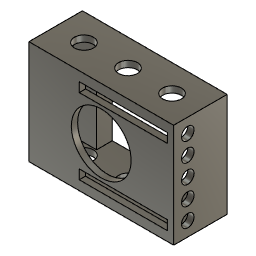
esp32 Box (Autodesk Fusion 360 design; units mm, degrees)
Autodesk Fusion 360 part; units mm, degrees
note: some values were not read from the file. Set by a fixed rule: which sketch regions a step uses.
sketch "Skizze1" plane through (0, 0, 0) normal (0, 1, 0) x (1, 0, 0)
  line L0 (0, 0) -> (46, 0)
  line L1 (46, 0) -> (46, -33)
  line L2 (46, -33) -> (0, -33)
  line L3 (0, -33) -> (0, 0)
  line L4 (2, -2) -> (44, -2)
  line L5 (44, -2) -> (44, -31)
  line L6 (44, -31) -> (2, -31)
  line L7 (2, -31) -> (2, -2)
  dimension "d1" = 46
  dimension "d2" = 33
  dimension "d3" = 2
  constraint horizontal L0
  constraint vertical L1
  constraint horizontal L2
  constraint vertical L3
  constraint coincident L0.start L3.end
  measures "d1" distance of L0.start L0.end
  measures "d2" distance of L0.start L2.end
extrude "Extrusion1" add sketch "Skizze1" against normal blind 2 contours L0 L1 L2 L3 | L4 L5 L6 L7
extrude "Extrusion2" add sketch "Skizze1" along normal blind 15
sketch "Skizze2" plane through (0, 0, 0) normal (0, 1, 0) x (1, 0, 0)
sketch "Skizze3" plane through (0, 15, 0) normal (0, 1, 0) x (-1, 0, 0)
  line L0 (-44, 31) -> (-2, 31)
  line L1 (-2, 31) -> (-2, 2)
  line L2 (-2, 2) -> (-44, 2)
  line L3 (-44, 2) -> (-44, 31)
  line L4 (0, 33) -> (-46, 33)
  line L5 (-46, 33) -> (-46, 0)
  line L6 (-46, 0) -> (0, 0)
  line L7 (0, 0) -> (0, 33)
  line L8 (-2, 31) -> (-9.5, 31)
  line L9 (-9.5, 31) -> (-9.5, 2)
  line L10 (-9.5, 2) -> (-2, 2)
  line L11 (-2, 2) -> (-2, 31)
  dimension "d8" = 7.5
  constraint horizontal L8
  constraint vertical L9
  constraint horizontal L10
  constraint vertical L11
  constraint coincident L0.end L1.start
  measures "d8" distance of L0.end L8.end
extrude "Extrusion3" add sketch "Skizze3" against normal blind 5 contours L0 L1 L2 L8 L9 L10 L11
sketch "Skizze4" plane through (0, -2, 0) normal (0, -1, 0) x (1, 0, 0)
  line L0 (46, 33) -> (0, 33)
  line L1 (0, 33) -> (0, 0)
  line L2 (0, 0) -> (46, 0)
  line L3 (46, 0) -> (46, 33)
  line L4 (46, 33) -> (16, 33)
  line L5 (16, 33) -> (16, 0)
  line L6 (16, 0) -> (46, 0)
  line L7 (46, 0) -> (46, 33)
  line L8 (16, 33) -> (46, 33)
  line L9 (16, 30) -> (16, 33)
  line L10 (16, 0) -> (46, 0)
  line L11 (46, 0) -> (46, 3)
  line L12 (46, 3) -> (16, 3)
  line L13 (16, 3) -> (16, 0)
  line L14 (16, 3) -> (46, 3)
  line L15 (46, 3) -> (46, 6)
  line L16 (46, 6) -> (16, 6)
  line L17 (16, 6) -> (16, 3)
  line L18 (0, 33) -> (46, 0)
  line L19 (46, 33) -> (0, 0)
  circle A0 centre (23, 16.5) radius 9.5
  line L20 (44, 35) -> (44, -3)
  line L21 (16, 30) -> (44, 30)
  line L22 (44, 30) -> (44, 27)
  line L23 (44, 27) -> (16, 27)
  line L24 (16, 27) -> (16, 30)
  dimension "d12" = 3
  constraint horizontal L4
  constraint vertical L5
  constraint horizontal L6
  constraint vertical L7
  constraint coincident L2 L5.end
  constraint coincident L0.start L3.end
  constraint horizontal L8
  constraint vertical L9
  constraint horizontal L10
  constraint vertical L11
  constraint horizontal L12
  constraint vertical L13
  constraint coincident L3 L11.end
  constraint horizontal L14
  constraint vertical L15
  constraint horizontal L16
  constraint vertical L17
  constraint coincident L0.end L1.start
  constraint coincident L1.end L2.start
  constraint midpoint L18 A0.centre
  constraint perpendicular L10 L20
  constraint horizontal L21
  constraint vertical L22
  constraint horizontal L23
  constraint vertical L24
  constraint coincident L20 L22.end
  measures "d12" distance of L12.end L16.end
extrude "Extrusion4" cut sketch "Skizze4" against normal blind 6 contours L5 L19 L21 L23 L24 | L5 L18 A0 | L5 L18 L19 A0 | L19 L20 L21 L22 L23 | L5 L19 A0 | L5 L18 L19 | L5 L18 L19 A0 | L5 L12 L14 L16 L17 L18 | L5 L18 L19 A0 | L18 L19 A0 | L12 L14 L16 L18 L20
sketch "Skizze5" plane through (0, 0, 0) normal (0, 0, -1) x (1, 0, 0)
  line L0 (46, -15) -> (46, 2)
  line L1 (46, 2) -> (0, 2)
  line L2 (0, 2) -> (0, -15)
  line L3 (0, -15) -> (46, -15)
  line L4 (46, -15) -> (0, 2)
  line L5 (46, 2) -> (0, -15)
  circle A0 centre (23, -6.5) radius 3
  circle A1 centre (9, -6.5) radius 3
  circle A2 centre (37, -6.5) radius 3
  dimension "d17" = 14
  dimension "d18" = 0
  dimension "d21" = 6
  constraint coincident L0.start L3.end
  constraint coincident L1.end L2.start
  constraint coincident L0.end L1.start
  constraint coincident L2.end L3.start
  constraint midpoint L5 A0.centre
  measures "d21" diameter of A0
extrude "Extrusion5" cut sketch "Skizze5" against normal blind 40 contours L4 L5 A0 | L4 L5 A0 | L4 L5 A0 | L4 L5 A0 | A1 | A2
sketch "Skizze6" plane through (0, 0, 0) normal (-1, 0, 0) x (0, -1, 0)
  line L0 (-15, 0) -> (2, 0)
  line L1 (2, 0) -> (2, 33)
  line L2 (2, 33) -> (-15, 33)
  line L3 (-15, 33) -> (-15, 0)
  line L4 (-15, 33) -> (2, 0)
  circle A0 centre (-6.5, 16.5) radius 2
  circle A1 centre (-2.5, 16.5) radius 2
  circle A2 centre (-2.5, 4.5) radius 2
  circle A3 centre (-2.5, 10.5) radius 2
  circle A4 centre (-2.5, 22.5) radius 2
  circle A5 centre (-2.5, 28.5) radius 2
  dimension "d22" = 4
  dimension "d25" = 4
  dimension "d26" = 0
  dimension "d29" = 0
  dimension "d30" = 12
  constraint coincident L2.end L3.start
  constraint coincident L0.end L1.start
  constraint midpoint L4 A0.centre
  measures "d22" diameter of A0
extrude "Extrusion6" cut sketch "Skizze6" against normal blind 130 contours A1 | L4 A2 | L4 A2 | L4 A3 | L4 A3 | A4 | A5
